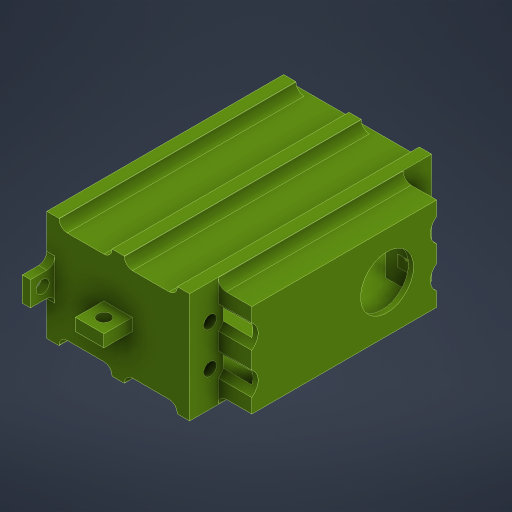
# Autodesk Inventor part: carcasa_servo
Saved by Autodesk Inventor 2023.1 (Build 271208000, 208)
## iProperties
Created: 2022-11-07
Part Number: carcasa_servo
Material: Generic
Document SubType Name: Modeling
Designer: amtat
Density: 1 g/cm^3
Appearance: Default
Author: amtat
Autodesk Inventor part; units mm, degrees
ref_plane "YZ Plane" through (0, 0, 0) normal (1, 0, 0) x (0, 1, 0)
ref_plane "XZ Plane" through (0, 0, 0) normal (0, 1, 0) x (-1, 0, 0)
ref_plane "XY Plane" through (0, 0, 0) normal (0, 0, 1) x (1, 0, 0)
sketch "Sketch1" plane through (0, 0, 0) normal (1, 0, 0) x (0, 1, 0)
  circle A0 centre (0, 0) radius 1.6
  circle A1 centre (10, 0) radius 1.6
  circle A2 centre (10, -49.2) radius 1.6
  circle A3 centre (0, -49.2) radius 1.6
  line L0 (10, 0) -> (10, -1.6)
  line L1 (10, -3.2) -> (0, -3.2)
  line L2 (10, -49.2) -> (10, -47.6)
  line L3 (10, -46) -> (0, -46)
  line L4 (10, -3.2) -> (5, -3.2)
  line L5 (5, -3.2) -> (15.15, -3.2)
  line L6 (15.15, -3.2) -> (15.15, -46)
  line L7 (15.15, -46) -> (-5.15, -46)
  line L8 (-5.15, -46) -> (-5.15, -3.2)
  line L9 (-5.15, -3.2) -> (5, -3.2)
  line L10 (0, 0) -> (0, -1.6)
  line L11 (0, -47.6) -> (0, -49.2)
  line L12 (0, 0) -> (1.6, 0)
  line L13 (8.4, 0) -> (10, 0)
  line L14 (0, -49.2) -> (1.6, -49.2)
  line L15 (8.4, -49.2) -> (10, -49.2)
  line L16 (15.15, -3.2) -> (16.4, -3.2)
  line L17 (16.4, -3.2) -> (16.4, -47.25)
  line L18 (16.4, -47.25) -> (-6.4, -47.25)
  line L19 (-6.4, -47.25) -> (-6.4, -1.95)
  line L20 (-6.4, -1.95) -> (16.4, -1.95)
  line L21 (16.4, -1.95) -> (16.4, -3.2)
  line L22 (10, 0) -> (10, -3.2)
  line L23 (10, -3.2) -> (10, 1.6)
  line L24 (10, 2.8) -> (16.4, 2.8)
  line L25 (16.4, 2.8) -> (16.4, -1.95)
  line L26 (10, 2.8) -> (-6.4, 2.8)
  line L27 (-6.4, 2.8) -> (-6.4, -1.95)
  line L28 (10, -49.2) -> (10, -46)
  line L29 (10, -46) -> (10, -52)
  line L30 (10, -52) -> (16.4, -52)
  line L31 (16.4, -52) -> (16.4, -47.25)
  line L32 (10, -52) -> (-6.4, -52)
  line L33 (-6.4, -52) -> (-6.4, -47.25)
  dimension "d0" = 3.2
  dimension "d1" = 10
  dimension "d2" = 3.2
  dimension "d3" = 49.2
  dimension "d4" = 3.2
  dimension "d5" = 3.2
  dimension "d6" = 3.2
  dimension "d7" = 3.2
  dimension "d8" = 5
  dimension "d9" = 10.15
  dimension "d10" = 20.3
  dimension "d11" = 1.25
  dimension "d12" = 44.05
  dimension "d13" = 22.8
  dimension "d14" = 45.3
  dimension "d15" = 6
  dimension "d16" = 6
  constraints: 68 end point, 22 perpendicular, 10 point on line, 9 point on circle, 5 vertical, 4 centre point, 4 coincident, 3 horizontal, 1 midpoint, 1 parallel
  measures "d0" diameter of A0
  measures "d1" distance of L10.start L13.end
  measures "d2" diameter of A1
  measures "d3" distance of L10.start L11.end
  measures "d4" diameter of A2
  measures "d5" diameter of A3
  measures "d6" distance of L0.start L1.start
  measures "d7" distance of L2.start L3.start
  measures "d8" distance of L1.start L4.end
  measures "d9" distance of L4.end L5.end
  measures "d10" distance of L6.end L7.end
  measures "d11" distance of L5.end L16.end
  measures "d12" distance of L16.end L17.end
  measures "d13" distance of L17.end L18.end
  measures "d14" distance of L18.end L19.end
  measures "d15" distance of L1.start L24.start
  measures "d16" distance of L3.start L29.end
extrude "Extrusion1" add sketch "Sketch1" along normal blind 3 contours A2 L28 L18 L31 L30 L29 | A2 L29 L32 L33 L18 L28 | L28 L7 L6 L16 L17 L18 | L18 L19 L20 L22 L1 L9 L8 L7 L3 L28 | L16 L5 L22 L20 L21 | L27 L26 L24 L25 L20
sketch "Sketch2" plane through (0, -6.4, 2.8) normal (0, 0, 1) x (1, 0, 0)
  line L0 (0, 22.8) -> (0, 0) projected
  line L1 (0, 0) -> (3, 0) projected
  line L2 (3, 22.8) -> (3, 0) projected
  line L3 (0, 22.8) -> (3, 22.8) projected
  point P0 (0, 6.4)
extrude "Extrusion2" add sketch "Sketch2" along normal blind 1
sketch "Sketch3" plane through (0, -6.4, -52) normal (0, 0, -1) x (-1, 0, 0)
  line L0 (0, 0) -> (0, 22.8) projected
  line L1 (0, 22.8) -> (-3, 22.8) projected
  line L2 (-3, 0) -> (-3, 22.8) projected
  line L3 (0, 0) -> (-3, 0) projected
  point P0 (0, 6.4)
extrude "Extrusion3" add sketch "Sketch3" along normal blind 1
sketch "Sketch4" plane through (3, 0, 0) normal (1, 0, 0) x (0, 0, -1)
  line L0 (53, -6.4) -> (-3.8, -6.4) projected
  line L1 (53, 16.4) -> (53, -6.4) projected
  line L2 (-3.8, 16.4) -> (53, 16.4) projected
  line L3 (-3.8, -6.4) -> (-3.8, 16.4) projected
  circle A0 centre (0, 10) radius 1.6 projected
  circle A1 centre (49.2, 0) radius 1.6 projected
  circle A2 centre (49.2, 10) radius 1.6 projected
  line L4 (3.2, -5.15) -> (3.2, 15.15) projected
  line L5 (3.2, 15.15) -> (46, 15.15) projected
  line L6 (46, 15.15) -> (46, -5.15) projected
  line L7 (46, -5.15) -> (3.2, -5.15) projected
  circle A3 centre (0, 0) radius 1.6 projected
  line L8 (3.2, 15.15) -> (46, 15.15) projected
  line L9 (3.2, 15.15) -> (3.2, 16.4)
  line L10 (3.2, 16.4) -> (1.95, 16.4)
  line L11 (-3.8, 16.4) -> (53, 16.4) projected
  line L12 (1.95, 16.4) -> (1.95, -6.4)
  line L13 (-3.8, -6.4) -> (53, -6.4) projected
  line L14 (46, 15.15) -> (46, -5.15) projected
  line L15 (46, 15.15) -> (46, 16.4)
  line L16 (46, 16.4) -> (47.25, 16.4)
  line L17 (47.25, 16.4) -> (47.25, -6.4)
  dimension "d23" = 1.25
  dimension "d24" = 1.25
  constraints: 12 end point, 6 point on line, 3 perpendicular, 1 collinear
  measures "d23" distance of L9.end L10.end
  measures "d24" distance of L15.end L16.end
extrude "Extrusion4" add sketch "Sketch4" along normal blind 7 contours L0 L12 L2 L9 L4 L7 L6 L15 L17 | L15 L5 L9 L2
sketch "Sketch5" plane through (10, 0, 0) normal (1, 0, 0) x (0, 0, -1)
  line L0 (1.95, 16.4) -> (1.95, -6.4) projected
  line L1 (1.95, -6.4) -> (47.25, -6.4) projected
  line L2 (47.25, -6.4) -> (47.25, 16.4) projected
  line L3 (47.25, 16.4) -> (1.95, 16.4) projected
  line L4 (46, 15.15) -> (46, -5.15) projected
  line L5 (46, -5.15) -> (3.2, -5.15) projected
  line L6 (3.2, -5.15) -> (3.2, 15.15) projected
  line L7 (3.2, 15.15) -> (46, 15.15) projected
  line L8 (47.25, 16.4) -> (47.25, -6.4) projected
  line L9 (53, -6.4) -> (47.25, -6.4) projected
  line L10 (53, 16.4) -> (53, -6.4) projected
  line L11 (47.25, 16.4) -> (53, 16.4) projected
  circle A0 centre (49.2, 0) radius 1.6 projected
  circle A1 centre (49.2, 10) radius 1.6 projected
  line L12 (49.2, 10) -> (49.2, 5)
  line L13 (49.2, 5) -> (35.1, 5)
  circle A2 centre (35.1, 5) radius 6.5
  point P0 (0, 0)
  dimension "d27" = 5
  dimension "d28" = 14.1
  dimension "d29" = 13
  constraints: 4 end point, 1 centre point, 1 coincident, 1 horizontal, 1 vertical
  measures "d27" distance of L12.start L12.end
  measures "d28" distance of L12.end L13.end
  measures "d29" diameter of A2
extrude "Extrusion5" add sketch "Sketch5" along normal blind 1.25 contours L3 L2 L1 L0 | L4 L5 L6 L7
sketch "Sketch6" plane through (0, -6.4, 3.8) normal (0, 0, 1) x (1, 0, 0)
  line L0 (0, 22.8) -> (0, 0) projected
  line L1 (0, 0) -> (3, 0) projected
  line L2 (3, 0) -> (3, 22.8) projected
  line L3 (3, 22.8) -> (0, 22.8) projected
  point P0 (0, 6.4)
extrude "Extrusion6" add sketch "Sketch6" along normal blind 1.25
sketch "Sketch7" plane through (0, -6.4, -53) normal (0, 0, -1) x (-1, 0, 0)
  line L0 (0, 0) -> (0, 22.8) projected
  line L1 (0, 22.8) -> (-3, 22.8) projected
  line L2 (-3, 22.8) -> (-3, 0) projected
  line L3 (-3, 0) -> (0, 0) projected
  point P0 (0, 6.4)
extrude "Extrusion7" add sketch "Sketch7" along normal blind 1.25
sketch "Sketch8" plane through (0, 0, 0) normal (-1, 0, 0) x (0, 0, 1)
  line L0 (5.05, -6.4) -> (-54.25, -6.4) projected
  line L1 (5.05, 16.4) -> (5.05, -6.4) projected
  line L2 (5.05, 16.4) -> (-54.25, 16.4) projected
  line L3 (-54.25, -6.4) -> (-54.25, 16.4) projected
  circle A0 centre (0, 10) radius 1.6 projected
  circle A1 centre (-49.2, 0) radius 1.6 projected
  circle A2 centre (-49.2, 10) radius 1.6 projected
  line L4 (-3.2, -5.15) -> (-3.2, 15.15) projected
  line L5 (-46, -5.15) -> (-3.2, -5.15) projected
  line L6 (-46, 15.15) -> (-46, -5.15) projected
  line L7 (-3.2, 15.15) -> (-46, 15.15) projected
  circle A3 centre (0, 0) radius 1.6 projected
  line L8 (5.05, -6.4) -> (-54.25, -6.4) projected
  line L9 (5.05, -6.4) -> (3.8, -6.4)
  line L10 (3.8, -6.4) -> (3.8, 16.4)
  line L11 (5.05, 16.4) -> (-54.25, 16.4) projected
  line L12 (-3.2, -5.15) -> (3.8, -5.15)
  line L13 (-3.2, 15.15) -> (-46, 15.15) projected
  line L14 (-3.2, 15.15) -> (3.8, 15.15)
  line L15 (-54.25, 16.4) -> (-53, 16.4)
  line L16 (-53, 16.4) -> (-53, -6.4)
  line L17 (-46, -5.15) -> (-3.2, -5.15) projected
  line L18 (-46, -5.15) -> (-53, -5.15)
  line L19 (-46, 15.15) -> (-53, 15.15)
  dimension "d36" = 1.25
  dimension "d37" = 1.25
  constraints: 16 end point, 10 point on line, 4 perpendicular
  measures "d36" distance of L0.start L9.end
  measures "d37" distance of L2.end L15.end
extrude "Extrusion8" add sketch "Sketch8" along normal blind 28 contours L0 L10 L2 L1 | L0 L16 L18 L5 L12 L10 | L0 L3 L2 L16 | L10 L14 L7 L19 L16 L2
sketch "Sketch9" plane through (11.25, 0, 0) normal (1, 0, 0) x (0, 0, -1)
  line L0 (47.25, 16.4) -> (47.25, -6.4) projected
  line L1 (54.25, -6.4) -> (47.25, -6.4) projected
  line L2 (54.25, 16.4) -> (54.25, -6.4) projected
  line L3 (47.25, 16.4) -> (54.25, 16.4) projected
  circle A0 centre (49.2, 0) radius 1.6 projected
  circle A1 centre (49.2, 10) radius 1.6 projected
  line L4 (1.95, -6.4) -> (1.95, 16.4) projected
  line L5 (-5.05, 16.4) -> (1.95, 16.4) projected
  line L6 (-5.05, -6.4) -> (-5.05, 16.4) projected
  line L7 (1.95, -6.4) -> (-5.05, -6.4) projected
  circle A2 centre (0, 10) radius 1.6 projected
  circle A3 centre (0, 0) radius 1.6 projected
  circle A4 centre (49.2, 0) radius 3.5
  circle A5 centre (49.2, 10) radius 3.5
  circle A6 centre (0, 0) radius 3.5
  circle A7 centre (0, 10) radius 3.5
  point P0 (1.95, 12.9065)
  point P1 (1.95, 7.0935)
  point P2 (1.95, 2.9065)
  point P3 (1.95, -2.9065)
  point P4 (47.25, 7.0935)
  point P5 (47.25, 12.9065)
  point P6 (47.25, -2.9065)
  point P7 (47.25, 2.9065)
  dimension "d40" = 7
  dimension "d41" = 7
  dimension "d42" = 7
  dimension "d43" = 7
  constraints: 4 centre point, 4 coincident
  measures "d40" diameter of A4
  measures "d41" diameter of A5
  measures "d42" diameter of A6
  measures "d43" diameter of A7
extrude "Extrusion9" cut sketch "Sketch9" against normal blind 8.25 contours L0 A5 | L0 A4 | L4 A6 | L4 A7 picked at (46.5526, 9.5305) picked at (46.5526, -0.4695) picked at (2.1656, 0.7823) picked at (2.1656, 10.7823)
sketch "Sketch10" plane through (3, 16.4, -1.95) normal (0, 1, 0) x (1, 0, 0)
  line L0 (0, -7) -> (-31, -7) projected
  line L1 (0, -7) -> (0, 0) projected
  line L2 (0, 0) -> (8.25, 0) projected
  line L3 (8.25, 45.3) -> (8.25, 0) projected
  line L4 (0, 45.3) -> (8.25, 45.3) projected
  line L5 (0, 45.3) -> (0, 52.3) projected
  line L6 (0, 52.3) -> (-31, 52.3) projected
  line L7 (-31, -7) -> (-31, 52.3) projected
  line L8 (0, 45.3) -> (0, 52.3) projected
  line L9 (0, 52.3) -> (-3, 52.3)
  line L10 (0, 52.3) -> (-31, 52.3) projected
  line L11 (-3, 52.3) -> (-3, -7)
  line L12 (0, 0) -> (0, 45.3)
  line L13 (0, -0.35) -> (0, -3.55) projected
  point P0 (-3, -1.95)
  dimension "d46" = 3
  constraints: 6 end point, 2 point on line, 1 collinear, 1 perpendicular
  measures "d46" distance of L5.end L9.end
extrude "Extrusion10" add sketch "Sketch10" along normal blind 1.75 contours L0 L11 L6 L5 L12 L1
sketch "Sketch11" plane through (3, -6.4, -47.25) normal (0, -1, 0) x (1, 0, 0)
  line L0 (0, 52.3) -> (0, -7) projected
  line L1 (0, -7) -> (-3, -7) projected
  line L2 (-3, -7) -> (-3, 52.3) projected
  line L3 (-3, 52.3) -> (0, 52.3) projected
  point P0 (-3, 47.25)
extrude "Extrusion11" add sketch "Sketch11" along normal blind 1.75
sketch "Sketch12" plane through (-28, 0, 0) normal (-1, 0, 0) x (0, 0, 1)
  line L0 (5.05, -6.4) -> (5.05, 16.4) projected
  line L1 (5.05, 16.4) -> (-54.25, 16.4) projected
  line L2 (-54.25, 16.4) -> (-54.25, -6.4) projected
  line L3 (-54.25, -6.4) -> (5.05, -6.4) projected
  line L4 (3.8, -5.15) -> (-53, -5.15) projected
  line L5 (-53, -5.15) -> (-53, 15.15) projected
  line L6 (-53, 15.15) -> (3.8, 15.15) projected
  line L7 (3.8, 15.15) -> (3.8, -5.15) projected
  point P0 (0, 0)
extrude "Extrusion12" add sketch "Sketch12" along normal blind 4
sketch "Sketch13" plane through (-32, 0, 0) normal (-1, 0, 0) x (0, 0, 1)
  line L0 (5.05, 16.4) -> (-54.25, 16.4) projected
  line L1 (-54.25, 16.4) -> (-54.25, -6.4) projected
  line L2 (-54.25, -6.4) -> (5.05, -6.4) projected
  line L3 (5.05, -6.4) -> (5.05, 16.4) projected
  line L4 (3.8, -5.15) -> (-53, -5.15) projected
  line L5 (-53, -5.15) -> (-53, 15.15) projected
  line L6 (-53, 15.15) -> (3.8, 15.15) projected
  line L7 (3.8, 15.15) -> (3.8, -5.15) projected
  line L8 (5.05, 16.4) -> (5.05, 5)
  line L9 (5.05, 5) -> (5.05, 8)
  line L10 (5.05, 18.15) -> (5.05, -8.15) projected
  line L11 (5.05, 8) -> (11.05, 8)
  line L12 (11.05, 8) -> (11.05, 2)
  line L13 (11.05, 2) -> (5.05, 2)
  line L14 (5.05, 5) -> (8.05, 5)
  circle A0 centre (8.05, 5) radius 1.6
  point P0 (0, 0)
  dimension "d54" = 11.4
  dimension "d55" = 3
  dimension "d56" = 6
  dimension "d57" = 6
  dimension "d58" = 3.2
  constraints: 12 end point, 3 perpendicular, 2 point on line, 1 centre point, 1 coincident, 1 horizontal, 1 midpoint
  measures "d54" distance of L0.start L8.end
  measures "d55" distance of L8.end L9.end
  measures "d56" distance of L9.end L11.end
  measures "d57" distance of L11.end L12.end
  measures "d58" diameter of A0
extrude "Extrusion13" add sketch "Sketch13" against normal blind 2 contours L11 L12 L13 L3
sketch "Sketch14" plane through (0, -6.4, 5.05) normal (0, 0, 1) x (1, 0, 0)
  line L0 (-30, 8.4) -> (-32, 8.4) projected
  line L1 (-32, 0) -> (-32, 8.4) projected
  line L2 (0, 0) -> (-32, 0) projected
  line L3 (3, -1.75) -> (0, -1.75) projected
  line L4 (3, 24.55) -> (3, -1.75) projected
  line L5 (0, 24.55) -> (3, 24.55) projected
  line L6 (0, 22.8) -> (-32, 22.8) projected
  line L7 (-32, 14.4) -> (-32, 22.8) projected
  line L8 (-32, 14.4) -> (-30, 14.4) projected
  line L9 (-30, 14.4) -> (-30, 8.4) projected
  line L10 (-1.9843, 22.8) -> (-32, 22.8) projected
  line L11 (-32, 22.8) -> (-14.5, 22.8)
  line L12 (-14.5, 22.8) -> (-14.5, 11.4)
  line L13 (-14.5, 11.4) -> (-14.5, 12.9)
  line L14 (-14.5, 12.9) -> (-11, 12.9)
  line L15 (-11, 12.9) -> (-11, 9.9)
  line L16 (-11, 9.9) -> (-18, 9.9)
  line L17 (-18, 9.9) -> (-18, 12.9)
  line L18 (-18, 12.9) -> (-14.5, 12.9)
  line L19 (0, 0) -> (0, -1.75) projected
  line L20 (0, 22.8) -> (0, 24.55) projected
  point P0 (0, 6.4)
  dimension "d61" = 17.5
  dimension "d62" = 11.4
  dimension "d63" = 1.5
  dimension "d64" = 3.5
  dimension "d65" = 3
  dimension "d66" = 7
  constraints: 16 end point, 6 perpendicular, 3 point on line
  measures "d61" distance of L6.end L11.end
  measures "d62" distance of L11.end L12.end
  measures "d63" distance of L12.end L13.end
  measures "d64" distance of L13.end L14.end
  measures "d65" distance of L14.end L15.end
  measures "d66" distance of L15.end L16.end
extrude "Extrusion14" add sketch "Sketch14" along normal blind 7 contours L14 L15 L16 L17 L18
sketch "Sketch15" plane through (-18, 6.5, 5.05) normal (0, 1, 0) x (1, 0, 0)
  line L0 (0, 0) -> (7, 0) projected
  line L1 (0, 0) -> (0, -7) projected
  line L2 (7, -7) -> (0, -7) projected
  line L3 (7, 0) -> (7, -7) projected
  line L4 (0, 0) -> (3.5, 0)
  line L5 (18, 0) -> (-14, 0) projected
  line L6 (3.5, 0) -> (3.5, -3.5)
  circle A0 centre (3.5, -3.5) radius 1.6
  point P0 (18, 5.05)
  point P1 (16.0157, 0)
  dimension "d69" = 3.5
  dimension "d70" = 3.5
  dimension "d71" = 3.2
  constraints: 4 end point, 1 centre point, 1 coincident, 1 perpendicular, 1 point on line
  measures "d69" distance of L0.start L4.end
  measures "d70" distance of L4.end L6.end
  measures "d71" diameter of A0
sketch "Sketch16" plane through (0, -6.4, -54.25) normal (0, 0, -1) x (-1, 0, 0)
  line L0 (18, 9.9) -> (11, 9.9) projected
  line L1 (11, 9.9) -> (11, 12.9) projected
  line L2 (11, 12.9) -> (18, 12.9) projected
  line L3 (18, 12.9) -> (18, 9.9) projected
  point P0 (0, 6.4)
extrude "Extrusion15" add sketch "Sketch16" along normal blind 7
sketch "Sketch17" plane through (-18, 6.5, -54.25) normal (0, 1, 0) x (1, 0, 0)
  point P0 (18, -54.25)
sketch "Sketch18" plane through (-18, 6.5, -54.25) normal (0, 1, 0) x (1, 0, 0)
  line L0 (7, 0) -> (0, 0) projected
  line L1 (7, 0) -> (7, 7) projected
  line L2 (0, 7) -> (7, 7) projected
  line L3 (0, 0) -> (0, 7) projected
  line L4 (0, 0) -> (7, 0) projected
  line L5 (7, 0) -> (3.5, 0)
  line L6 (3.5, 0) -> (3.5, 3.5)
  circle A0 centre (3.5, 3.5) radius 1.6
  circle A1 centre (3.5, -62.8) radius 1.6 projected
  point P0 (18, -54.25)
  dimension "d74" = 3.5
  dimension "d75" = 3.5
  dimension "d76" = 3.2
  constraints: 4 end point, 1 centre point, 1 coincident, 1 midpoint, 1 perpendicular
  measures "d74" distance of L0.start L5.end
  measures "d75" distance of L5.end L6.end
  measures "d76" diameter of A0
extrude "Extrusion16" cut sketch "Sketch18" against normal blind 7 contours A0 | A1
sketch "Sketch19" plane through (3, -8.15, -47.25) normal (0, -1, 0) x (1, 0, 0)
  line L0 (-3, 52.3) -> (-3, -7) projected
  line L1 (-3, -7) -> (0, -7) projected
  line L2 (0, -7) -> (0, 52.3) projected
  line L3 (0, 52.3) -> (-3, 52.3) projected
  point P0 (-3, 47.25)
extrude "Extrusion17" add sketch "Sketch19" along normal blind 0.35
sketch "Sketch20" plane through (3, 18.15, -1.95) normal (0, 1, 0) x (1, 0, 0)
  line L0 (0, -7) -> (0, 52.3) projected
  line L1 (0, 52.3) -> (-3, 52.3) projected
  line L2 (-3, 52.3) -> (-3, -7) projected
  line L3 (-3, -7) -> (0, -7) projected
  point P0 (-3, -1.95)
extrude "Extrusion18" add sketch "Sketch20" along normal blind 0.35
sketch "Sketch21" plane through (0, 16.4, 5.05) normal (0, 1, 0) x (1, 0, 0)
  line L0 (0, 0) -> (0, 59.3) projected
  line L1 (0, 59.3) -> (-32, 59.3) projected
  line L2 (-32, 0) -> (-32, 59.3) projected
  line L3 (0, 0) -> (-32, 0) projected
  line L4 (3, 0) -> (3, 59.3) projected
  line L5 (0, 59.3) -> (0, 0) projected
  line L6 (-32, 59.3) -> (-32, 0) projected
  line L7 (-32, 0) -> (-32, 59.3)
  line L8 (-32, 59.3) -> (-29, 59.3)
  line L9 (0, 59.3) -> (-32, 59.3) projected
  line L10 (-29, 59.3) -> (-29, 0)
  line L11 (0, 0) -> (-32, 0) projected
  line L12 (-29, 0) -> (-16, 0)
  line L13 (-16, 0) -> (-13, 0)
  line L14 (-13, 0) -> (-13, 59.3)
  line L15 (-13, 59.3) -> (-16, 59.3)
  line L16 (0, 58.05) -> (-32, 58.05) projected
  line L17 (-16, 59.3) -> (-16, 0)
  point P0 (0, 5.05)
  point P1 (-29, 58.05)
  point P2 (-29, 0)
  point P3 (-16, 58.05)
  point P4 (-13, 58.05)
  dimension "d84" = 3
  dimension "d85" = 13
  dimension "d86" = 3
  constraints: 16 end point, 4 point on line, 2 midpoint, 2 perpendicular, 1 vertical
  measures "d84" distance of L1.end L8.end
  measures "d85" distance of L10.end L12.end
  measures "d86" distance of L12.end L13.end
extrude "Extrusion19" add sketch "Sketch21" along normal blind 2.1 contours L3 L17 L16 L14 | L3 L2 L16 L10
sketch "Sketch22" plane through (0, -6.4, -54.25) normal (0, -1, 0) x (1, 0, 0)
  line L0 (-16, 59.3) -> (-13, 59.3) projected
  line L1 (-13, 59.3) -> (-13, 1.25) projected
  line L2 (-13, 1.25) -> (-16, 1.25) projected
  line L3 (-16, 1.25) -> (-16, 59.3) projected
  line L4 (-32, 1.25) -> (-32, 59.3) projected
  line L5 (-32, 59.3) -> (-29, 59.3) projected
  line L6 (-29, 59.3) -> (-29, 1.25) projected
  line L7 (-29, 1.25) -> (-32, 1.25) projected
  point P0 (0, 54.25)
extrude "Extrusion20" add sketch "Sketch22" along normal blind 2.1
fillet "Fillet3" radius 2 2 edges at (-31, 8, 5.05) (-31, 2, 5.05)
fillet "Fillet4" radius 2 10 edges at (-29, 16.4, -23.975) (-13, 16.4, -23.975) (-16, 16.4, -23.975) (0, 16.4, -24.6) (3, 16.4, -24.6) (3, -6.4, -24.6) (-16, -6.4, -23.975) (0, -6.4, -24.6) (-13, -6.4, -23.975) (-29, -6.4, -23.975)
body "Solid1"
